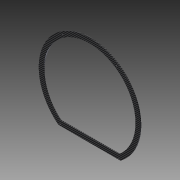
# Autodesk Inventor part: Handle Ring
Saved by Autodesk Inventor 2015 (Build 190159000, 159)
## iProperties
Created: 2016-09-21
Part Number: Handle Ring
Material: Generic
Document SubType Name: Modeling
Designer: James Yelland
Density: 1 g/cm^3
Appearance: Default
Author: James Yelland
Autodesk Inventor part; units mm, degrees
ref_plane "YZ Plane" through (0, 0, 0) normal (1, 0, 0) x (0, 1, 0)
ref_plane "XZ Plane" through (0, 0, 0) normal (0, 1, 0) x (-1, 0, 0)
ref_plane "XY Plane" through (0, 0, 0) normal (0, 0, 1) x (1, 0, 0)
sketch "Sketch1" plane through (0, 0, 0) normal (0, 1, 0) x (-1, 0, 0)
  line L0 (0, -83) -> (62.9285, -83)
  line L1 (0, -83) -> (-62.9285, -83)
  line L2 (0, -73) -> (59.3296, -73)
  line L3 (0, -73) -> (-59.3296, -73)
  arc A0 (65.4207, -82.1287) -> (-65.4207, -82.1287) centre (0, 0) ccw
  arc A1 (61.9375, -72.033) -> (-61.9375, -72.033) centre (0, 0) ccw
  arc A2 (59.3296, -73) -> (61.9375, -72.033) centre (59.3296, -69) ccw
  arc A3 (62.9285, -83) -> (65.4207, -82.1287) centre (62.9285, -79) ccw
  arc A4 (-65.4207, -82.1287) -> (-62.9285, -83) centre (-62.9285, -79) ccw
  arc A5 (-61.9375, -72.033) -> (-59.3296, -73) centre (-59.3296, -69) ccw
  circle A6 centre (60.1815, -79.8636) radius 1.6
  circle A7 centre (55.557, 83.147) radius 1.6
  circle A8 centre (-55.557, 83.147) radius 1.6
  circle A9 centre (-60.1815, -79.8636) radius 1.6
  point P0 (64.3117, -83)
  point P1 (-64.3117, -83)
  point P2 (60.7947, -73)
  point P3 (-60.7947, -73)
  dimension "d3" = 10
  dimension "d4" = 4
  dimension "d5" = 3.2
  dimension "d6" = 3.2
  constraints: 16 point on circle, 10 centre point, 8 end point, 8 tangent, 4 point on line, 3 equal radius, 2 coincident, 2 horizontal
  measures "d3" distance of L0.start L2.start
  measures "d4" radius of A2
  measures "d5" diameter of A6
  measures "d6" diameter of A7
extrude "Extrusion1" add sketch "Sketch1" along normal blind 2
body "Solid1"
